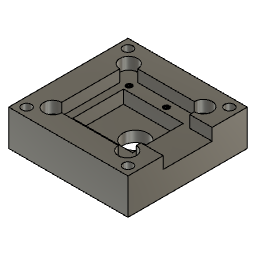
RaspPicam v3 (Autodesk Fusion 360 design; units mm, degrees)
Autodesk Fusion 360 part; units mm, degrees
sketch "Sketch1" plane through (0, 0, 0) normal (0, 0, 1) x (1, 0, 0)
  line L0 (20, 20) -> (-20, 20)
  line L1 (-20, 20) -> (-20, -20)
  line L2 (-20, -20) -> (20, -20)
  line L3 (20, -20) -> (20, 20)
  line L4 (20, 20) -> (-20, -20) construction
  line L5 (-20, 20) -> (20, -20) construction
  line L6 (17, 17) -> (-17, -17) construction
  line L7 (-17, 17) -> (17, -17) construction
  circle A0 centre (-17, -17) radius 1.6
  circle A1 centre (-17, 17) radius 1.6
  circle A2 centre (17, -17) radius 1.6
  circle A3 centre (17, 17) radius 1.6
  line L8 (17, -17) -> (17, -15.4)
  dimension "d1" = 40
  dimension "d2" = 40
  dimension "d3" = 34
  dimension "d4" = 34
  dimension "d5" = 3.2
  dimension "d6" = 3.2
  dimension "d7" = 3.2
  dimension "d8" = 3.2
  constraint horizontal L0
  constraint perpendicular L0 L1
  constraint parallel L0 L2
  constraint parallel L1 L3
  constraint coincident L4 origin
  constraint coincident L5 origin
  constraint coincident L6 origin
  constraint coincident L7 origin
  constraint coincident L6.end A0.centre
  constraint coincident L7.start A1.centre
  constraint coincident L7.end A2.centre
  constraint coincident L6.start A3.centre
  constraint coincident A2 L8.end
  measures "d1" distance of L1.end L2.end
  measures "d2" distance of L0.end L1.end
  measures "d3" distance of L6.end L7.end
  measures "d4" distance of L7.start L6.end
  measures "d5" diameter of A0
  measures "d6" diameter of A1
  measures "d7" diameter of A2
  measures "d8" diameter of A3
extrude "Extrude1" add sketch "Sketch1" against normal blind 12
sketch "Sketch2" plane through (0, 0, 0) normal (0, 0, 1) x (-1, 0, 0)
  circle A0 centre (17, 17) radius 1.6
  circle A1 centre (-17, -17) radius 1.6
  circle A2 centre (17, -17) radius 1.6
  circle A3 centre (-17, 17) radius 1.6
  line L0 (-20, 20) -> (-20, -20)
  line L1 (-20, -20) -> (20, -20)
  line L2 (20, -20) -> (20, 20)
  line L3 (20, 20) -> (-20, 20)
  line L4 (12.5, -12.75) -> (-12.5, -12.75)
  line L5 (-12.5, -12.75) -> (-12.5, 12.75)
  line L6 (-12.5, 12.75) -> (12.5, 12.75)
  line L7 (12.5, 12.75) -> (12.5, -12.75)
  line L8 (12.5, -12.75) -> (-12.5, 12.75) construction
  line L9 (-12.5, -12.75) -> (12.5, 12.75) construction
  line L10 (-12.5, 0) -> (-20, 0)
  line L11 (-12.5, -8.2) -> (-20, -8.2)
  line L12 (-20, -8.2) -> (-20, 8.2)
  line L13 (-20, 8.2) -> (-12.5, 8.2)
  line L14 (-12.5, 8.2) -> (-12.5, -8.2)
  line L15 (-12.5, -8.2) -> (-20, 8.2) construction
  line L16 (-20, -8.2) -> (-12.5, 8.2) construction
  point P0 (-16.25, 0)
  dimension "d11" = 25
  dimension "d12" = 25.5
  dimension "d13" = 16.4
  constraint horizontal L4
  constraint perpendicular L4 L5
  constraint parallel L4 L6
  constraint parallel L5 L7
  constraint coincident L8 origin
  constraint coincident L9 origin
  constraint midpoint L5 L10.start
  constraint midpoint L0 L10.end
  constraint horizontal L11
  constraint perpendicular L11 L12
  constraint parallel L11 L13
  constraint parallel L12 L14
  constraint coincident L15 P0
  constraint coincident L16 P0
  constraint midpoint L10 P0
  measures "d11" distance of L5.end L6.end
  measures "d12" distance of L4.end L5.end
  measures "d13" distance of L11.end L12.end
extrude "Extrude2" cut sketch "Sketch2" against normal blind 4 contours L0 L5 L10 L12 L13 L14 | L0 L5 L10 L11 L12 L14 | L4 L5 L6 L7 L14
sketch "Sketch3" plane through (0, 0, 0) normal (0, 0, 1) x (1, 0, 0)
  line L0 (0, 0) -> (2.5, 0)
  circle A0 centre (2.5, 0) radius 4.2
  dimension "d16" = 2.5
  dimension "d17" = 8.4
  constraint horizontal L0
  constraint coincident L0.start origin
  constraint coincident L0.end A0.centre
  measures "d16" distance of L0.start L0.end
  measures "d17" diameter of A0
extrude "Extrude3" cut sketch "Sketch3" against normal blind 16
sketch "Sketch4" plane through (0, 0, 0) normal (0, 0, 1) x (1, 0, 0)
  line L0 (-10, 8.5) -> (10, 8.5)
  line L1 (10, 8.5) -> (10, -8.5)
  line L2 (10, -8.5) -> (-10, -8.5)
  line L3 (-10, -8.5) -> (-10, 8.5)
  line L4 (-10, 8.5) -> (10, -8.5) construction
  line L5 (10, 8.5) -> (-10, -8.5) construction
  dimension "d20" = 20
  dimension "d21" = 17
  constraint horizontal L0
  constraint perpendicular L0 L1
  constraint parallel L0 L2
  constraint parallel L1 L3
  constraint coincident L4 origin
  constraint coincident L5 origin
  measures "d20" distance of L1.end L2.end
  measures "d21" distance of L0.end L1.end
extrude "Extrude4" cut sketch "Sketch4" against normal blind 8.4
sketch "Sketch5" plane through (0, 0, 0) normal (0, 0, 1) x (1, 0, 0)
  line L0 (-20, 20) -> (20, 20)
  line L1 (0, 0) -> (-3.75, 0)
  line L2 (2.5, 10.5) -> (-10, -10.5) construction
  line L3 (-10, 10.5) -> (2.5, -10.5) construction
  circle A0 centre (2.5, -10.5) radius 0.8
  circle A1 centre (-10, -10.5) radius 0.8
  circle A2 centre (-10, 10.5) radius 0.8
  circle A3 centre (2.5, 10.5) radius 0.8
  point P0 (-3.75, 0)
  dimension "d24" = 3.75
  dimension "d25" = 12.5
  dimension "d26" = 21
  dimension "d27" = 1.6
  dimension "d28" = 1.6
  dimension "d29" = 1.6
  dimension "d30" = 1.6
  constraint coincident L1.start origin
  constraint parallel L0 L1
  constraint coincident L2 P0
  constraint coincident L3 P0
  constraint coincident P0 L1.end
  constraint coincident L3.end A0.centre
  constraint coincident L2.end A1.centre
  constraint coincident L3.start A2.centre
  constraint coincident L2.start A3.centre
  measures "d24" distance of L1.start P0
  measures "d25" distance of L2.end L3.end
  measures "d26" distance of L3.start L2.end
  measures "d27" diameter of A0
  measures "d28" diameter of A1
  measures "d29" diameter of A2
  measures "d30" diameter of A3
extrude "Extrude5" cut sketch "Sketch5" against normal blind 18
sketch "Sketch6" plane through (0, 0, 0) normal (0, 0, 1) x (1, 0, 0)
  circle A0 centre (-12.5, -12.75) radius 3
  circle A1 centre (-12.5, 12.75) radius 3
  circle A2 centre (12.5, -12.75) radius 3
  circle A3 centre (12.5, 12.75) radius 3
  point P0 (-12.5, -12.75)
  point P1 (-12.5, 12.75)
  point P2 (12.5, -12.75)
  point P3 (12.5, 12.75)
  dimension "d33" = 6
  dimension "d34" = 6
  dimension "d35" = 6
  dimension "d36" = 6
  constraint coincident P0 A0.centre
  constraint coincident P1 A1.centre
  constraint coincident P2 A2.centre
  constraint coincident P3 A3.centre
  measures "d33" diameter of A0
  measures "d34" diameter of A1
  measures "d35" diameter of A2
  measures "d36" diameter of A3
extrude "Extrude6" cut sketch "Sketch6" against normal blind 4
thread "Thread1" "ISO Metric profile 2.0 M2x0.4 6H" major diameter 2.074 minor diameter 1.623 pitch 0.4 angle 60 modelled right hand crest width 0.1065 on face at (-9.204, -10.4203, -6.6667) crest through (-9.1885, -10.5, -4.1) on face at (-9.201, 10.4601, -9.3333) crest through (-9.1885, 10.5, -4.1) on face at (3.296, 10.4203, -9.3333) crest through (3.3115, 10.5, -4.1) on face at (3.296, -10.5797, -9.3333) crest through (3.3115, -10.5, -4.1)
